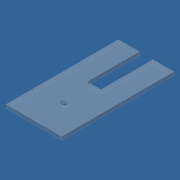
# Autodesk Inventor part: S1702_replat
Saved by Autodesk Inventor 2015 SP2 (Build 190223200, 223)
## iProperties
Created: 2017-10-30
Part Number: S1702_replat
Project: S1702_Circuit_Course
Material: Plastique PMMA
Description: Replat
Document SubType Name: Modeling
Designer: Benoit.CURCHOD2
Authority: 140X48x3
Density: 1.188 g/cm^3
Appearance: Transparent - Clair
Mass: 14.63 g
Surface Area: 93.8088 cm^2
Volume: 12.3148 cm^3
Material number: ---
Author: Benoit.CURCHOD2
Autodesk Inventor part; units mm, degrees
ref_plane "Plan YZ" through (0, 0, 0) normal (1, 0, 0) x (0, 1, 0)
ref_plane "Plan XZ" through (0, 0, 0) normal (0, 1, 0) x (-1, 0, 0)
ref_plane "Plan XY" through (0, 0, 0) normal (0, 0, 1) x (1, 0, 0)
sketch "Esquisse6" plane through (0, 0, 0) normal (0, 0, 1) x (1, 0, 0)
  line L0 (0, -20) -> (0, 120) construction
  line L1 (-24, 0) -> (24, 0)
  line L2 (24, 0) -> (24, 100)
  line L3 (24, 100) -> (6, 100)
  line L4 (6, 100) -> (6, 55)
  line L5 (6, 55) -> (-6, 55)
  line L6 (-6, 55) -> (-6, 100)
  line L7 (-6, 100) -> (-24, 100)
  line L8 (-24, 100) -> (-24, 0)
  line L9 (-33.6, 0) -> (33.6, 0) construction
  point P0 (0, 0)
  dimension "d0" = 100
  dimension "d1" = 48
  dimension "d2" = 12
  dimension "d3" = 45
  constraints: 16 end point, 5 perpendicular, 2 point on line, 1 collinear, 1 horizontal, 1 vertical, 2 other
  measures "d0" distance of L1.end L2.end
  measures "d1" distance of L1.start L1.end
  measures "d2" distance between parallel lines of L4 L6
  measures "d3" distance of L3.end L4.end
extrude "Extrusion1" add sketch "Esquisse6" along normal blind 3
sketch "Esquisse7" plane through (0, 0, 0) normal (0, 0, -1) x (-1, 0, 0)
  line L0 (0, -20) -> (0, 120) construction
  circle A0 centre (0, 30) radius 1.6
  line L1 (-24, 0) -> (24, 0) projected
  point P0 (0, 0)
  dimension "d8" = 3.2
  dimension "d9" = 30
  constraints: 1 centre point, 1 point on line
  measures "d8" diameter of A0
  measures "d9" distance from line of L1 A0.centre
extrude "Extrusion2" cut sketch "Esquisse7" against normal through all
chamfer "Chanfrein3" distance 1.8 angle 45 1 edges at (1.6, 30, 3)
sketch "Esquisse8" plane through (0, 0, 3) normal (0, 0, 1) x (1, 0, 0)
  line L0 (24, 100) -> (24, 0) projected
  line L1 (-24, 0) -> (24, 0)
  line L2 (24, 0) -> (24, 3)
  line L3 (24, 3) -> (-24, 3)
  line L4 (-24, 3) -> (-24, 0)
  line L5 (-24, 100) -> (-24, 0) projected
  line L6 (24, 0) -> (24, 100) projected
  line L7 (-24, 0) -> (24, 0) projected
  point P0 (0, 0)
  dimension "d21" = 3
  constraints: 8 end point, 2 collinear, 2 parallel, 1 horizontal, 1 perpendicular, 1 point on line
  measures "d21" distance between parallel lines of L3 L1
extrude "Extrusion3" cut sketch "Esquisse8" against normal through all
